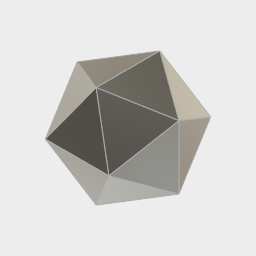
d20 v2 (Autodesk Fusion 360 design; units mm, degrees)
Autodesk Fusion 360 part; units mm, degrees
sketch "Sketch1" plane through (0, 0, 0) normal (0, 0, 1) x (1, 0, 0)
  line L0 (12.5, 20) -> (-12.5, 20)
  line L1 (-12.5, 20) -> (-12.5, -20)
  line L2 (-12.5, -20) -> (12.5, -20)
  line L3 (12.5, -20) -> (12.5, 20)
  line L4 (12.5, 20) -> (-12.5, -20) construction
  line L5 (-12.5, 20) -> (12.5, -20) construction
  dimension "d3" = 25
  dimension "d4" = 40
  measures "d3" distance of L1.end L2.end
  measures "d4" distance of L0.end L1.end
sketch "Sketch2" plane through (0, 0, 0) normal (0, 1, 0) x (1, 0, 0)
  line L0 (-20, -12.5) -> (20, -12.5)
  line L1 (20, -12.5) -> (20, 12.5)
  line L2 (20, 12.5) -> (-20, 12.5)
  line L3 (-20, 12.5) -> (-20, -12.5)
  line L4 (-20, -12.5) -> (20, 12.5) construction
  line L5 (20, -12.5) -> (-20, 12.5) construction
  dimension "d5" = 40
  dimension "d6" = 25
  measures "d5" distance of L1.end L2.end
  measures "d6" distance of L0.end L1.end
sketch "Sketch3" plane through (0, 0, 0) normal (1, 0, 0) x (0, 1, 0)
  line L0 (-12.5, 20) -> (12.5, 20)
  line L1 (12.5, 20) -> (12.5, -20)
  line L2 (12.5, -20) -> (-12.5, -20)
  line L3 (-12.5, -20) -> (-12.5, 20)
  line L4 (-12.5, 20) -> (12.5, -20) construction
  line L5 (12.5, 20) -> (-12.5, -20) construction
  dimension "d7" = 40
  dimension "d8" = 25
  measures "d7" distance of L0.end L1.end
  measures "d8" distance of L1.end L2.end
sketch "Sketch4" plane through (0, 0, 0) normal (0, 0, 1) x (1, 0, 0)
  line L0 (20, 0, 12.5) -> (0, 12.5, 20)
  line L1 (0, 12.5, 20) -> (12.5, 20, 0)
  line L2 (12.5, 20, 0) -> (20, 0, 12.5)
  line L3 (20, 0, 12.5) -> (0, -12.5, 20)
  line L4 (0, -12.5, 20) -> (0, 12.5, 20)
  line L5 (12.5, -20, 0) -> (0, -12.5, 20)
  line L6 (12.5, -20, 0) -> (20, 0, 12.5)
  line L7 (-12.5, -20, 0) -> (0, -12.5, 20)
  line L8 (-12.5, -20) -> (12.5, -20)
  line L9 (-20, 0, 12.5) -> (0, -12.5, 20)
  line L10 (-20, 0, 12.5) -> (-12.5, -20, 0)
  line L11 (0, 12.5, 20) -> (-20, 0, 12.5)
  line L12 (12.5, 20) -> (-12.5, 20)
  line L13 (0, 12.5, 20) -> (-12.5, 20, 0)
  line L14 (-12.5, 20, 0) -> (-20, 0, 12.5)
  line L15 (12.5, -20, 0) -> (20, 0, -12.5)
  line L16 (20, 0, -12.5) -> (12.5, 20, 0)
  line L17 (20, 0, 12.5) -> (20, 0, -12.5)
  line L18 (-12.5, 20, 0) -> (-20, 0, -12.5)
  line L19 (-20, 0, -12.5) -> (-12.5, -20, 0)
  line L20 (-20, 0, 12.5) -> (-20, 0, -12.5)
  line L21 (-20, 0, -12.5) -> (0, -12.5, -20)
  line L22 (0, -12.5, -20) -> (-12.5, -20, 0)
  line L23 (0, -12.5, -20) -> (12.5, -20, 0)
  line L24 (0, -12.5, -20) -> (20, 0, -12.5)
  line L25 (0, -12.5, -20) -> (0, 12.5, -20)
  line L26 (0, 12.5, -20) -> (-20, 0, -12.5)
  line L27 (0, 12.5, -20) -> (12.5, 20, 0)
  line L28 (0, 12.5, -20) -> (-12.5, 20, 0)
  line L29 (20, 0, -12.5) -> (0, 12.5, -20)
  point P0 (20, 0)
  point P1 (0, 12.5)
  point P2 (12.5, 20)
  point P3 (0, -12.5)
  point P4 (12.5, -20)
  point P5 (-12.5, -20)
  point P6 (-20, 0)
  point P7 (-12.5, 20)
  point P8 (20, 0)
  point P9 (-20, 0)
  point P10 (0, -12.5)
  point P11 (0, 12.5)
extrude "Extrude1" add sketch "Sketch4" against normal blind 1 contours L0 L1 L2 in plane through (10.8333, 10.8333, 10.8333) normal (0.57735, 0.57735, 0.57735)
extrude "Extrude2" add sketch "Sketch4" against normal blind 1 contours L2 L16 L17 in plane through (17.5342, 6.5753, 0) normal (0.936329, 0.351123, 0)
extrude "Extrude3" add sketch "Sketch4" against normal blind 1 contours L6 L15 L17 in plane through (17.5342, -6.5753, 0) normal (0.936329, -0.351123, 0)
extrude "Extrude4" add sketch "Sketch4" against normal blind 1 contours L0 L3 L4 in plane through (6.5753, 0, 17.5342) normal (0.351123, 0, 0.936329)
extrude "Extrude5" add sketch "Sketch4" against normal blind 1 contours L3 L5 L6 in plane through (10.8333, -10.8333, 10.8333) normal (0.57735, -0.57735, 0.57735)
extrude "Extrude6" add sketch "Sketch4" along normal blind 1 contours L5 L7 L8 in plane through (0, -17.5342, 6.5753) normal (0, 0.936329, -0.351123)
extrude "Extrude7" add sketch "Sketch4" along normal blind 1 contours L7 L9 L10 in plane through (-10.8333, -10.8333, 10.8333) normal (0.57735, 0.57735, -0.57735)
extrude "Extrude8" add sketch "Sketch4" against normal blind 1 contours L4 L9 L11 in plane through (-6.5753, 0, 17.5342) normal (-0.351123, 0, 0.936329)
extrude "Extrude9" add sketch "Sketch4" against normal blind 1 contours L11 L13 L14 in plane through (-10.8333, 10.8333, 10.8333) normal (-0.57735, 0.57735, 0.57735)
extrude "Extrude10" add sketch "Sketch4" along normal blind 1 contours L14 L18 L20 in plane through (-17.5342, 6.5753, 0) normal (0.936329, -0.351123, 0)
extrude "Extrude11" add sketch "Sketch4" along normal blind 1 contours L10 L19 L20 in plane through (-17.5342, -6.5753, 0) normal (0.936329, 0.351123, 0)
extrude "Extrude12" add sketch "Sketch4" against normal blind 1 contours L1 L12 L13 in plane through (0, 17.5342, 6.5753) normal (0, 0.936329, 0.351123)
extrude "Extrude13" add sketch "Sketch4" against normal blind 1 contours L16 L27 L29 in plane through (10.8333, 10.8333, -10.8333) normal (0.57735, 0.57735, -0.57735)
extrude "Extrude14" add sketch "Sketch4" against normal blind 1 contours L12 L27 L28 in plane through (0, 17.5342, -6.5753) normal (0, 0.936329, -0.351123)
extrude "Extrude15" add sketch "Sketch4" along normal blind 1 contours L18 L26 L28 in plane through (-10.8333, 10.8333, -10.8333) normal (0.57735, -0.57735, 0.57735)
extrude "Extrude16" add sketch "Sketch4" along normal blind 1 contours L24 L25 L29 in plane through (6.5753, 0, -17.5342) normal (-0.351123, 0, 0.936329)
extrude "Extrude17" add sketch "Sketch4" along normal blind 1 contours L21 L25 L26 in plane through (-6.5753, 0, -17.5342) normal (0.351123, 0, 0.936329)
extrude "Extrude18" add sketch "Sketch4" against normal blind 1 contours L15 L23 L24 in plane through (10.8333, -10.8333, -10.8333) normal (0.57735, -0.57735, -0.57735)
extrude "Extrude19" add sketch "Sketch4" along normal blind 1 contours L19 L21 L22 in plane through (-10.8333, -10.8333, -10.8333) normal (0.57735, 0.57735, 0.57735)
extrude "Extrude20" add sketch "Sketch4" along normal blind 1 contours L8 L22 L23 in plane through (0, -17.5342, -6.5753) normal (0, 0.936329, 0.351123)
